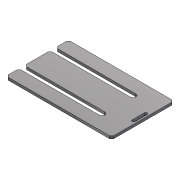
# Autodesk Inventor part: BC-10027
Saved by Autodesk Inventor 2016 (Build 200138000, 138)
## iProperties
Created: 2016-06-03
Part Number: BC-10027
Project: DIPOLO BC-3T- SIRIUS
Cost Center: 1504002005
Material: Aço Inox AISI 316
Document SubType Name: Modeling
Designer: reinaldo.basilio
Density: 7.85483 g/cm^3
Appearance: Semi-Polished
Description: Calço de ajuste da altura dos compensadores de gradiente.
Mass: 113.287 g
Surface Area: 128.736 cm^2
Volume: 14.4227 cm^3
RuleStatus: InUse
DocNumber: XXXXX-XXX-XXXX-00-001.ipt
Folder: .
Title: DIPOLO BC-3T- SIRIUS
Author: reinaldo.basilio
Autodesk Inventor part; units mm, degrees
ref_plane "YZ Plane" through (0, 0, 0) normal (1, 0, 0) x (0, 1, 0)
ref_plane "XZ Plane" through (0, 0, 0) normal (0, 1, 0) x (-1, 0, 0)
ref_plane "XY Plane" through (0, 0, 0) normal (0, 0, 1) x (1, 0, 0)
sketch "Sketch5" plane through (0, 0, 0) normal (0, 0, 1) x (1, 0, 0)
  line L0 (-31, 52.5) -> (31, 52.5)
  line L1 (31, 52.5) -> (31, -52.5)
  line L2 (-31, -52.5) -> (-31, 52.5)
  line L3 (-15.5, 27.5) -> (-15.5, -52.5) construction
  line L4 (-18.25, 27.5) -> (-18.25, -52.5)
  line L5 (-12.75, -52.5) -> (-12.75, 27.5)
  arc A0 (-12.75, 27.5) -> (-18.25, 27.5) centre (-15.5, 27.5) ccw
  arc A1 (-18.25, -52.5) -> (-12.75, -52.5) centre (-15.5, -52.5) ccw
  line L6 (0, 0) -> (0, 14.7878) construction
  line L7 (15.5, 27.5) -> (15.5, -52.5) construction
  line L8 (18.25, 27.5) -> (18.25, -52.5)
  line L9 (12.75, -52.5) -> (12.75, 27.5)
  arc A2 (18.25, 27.5) -> (12.75, 27.5) centre (15.5, 27.5) ccw
  arc A3 (12.75, -52.5) -> (18.25, -52.5) centre (15.5, -52.5) ccw
  line L10 (-18.25, -52.5) -> (-31, -52.5)
  line L11 (31, -52.5) -> (18.25, -52.5)
  line L12 (12.75, -52.5) -> (-12.75, -52.5)
  point P0 (0, 52.5)
  point P1 (-31, 0)
  point P2 (-15.5, -12.5)
  dimension "d8" = 62
  dimension "d9" = 105
  dimension "d10" = 15.5
  dimension "d11" = 5.5
  dimension "d12" = 80
  constraints: 30 end point, 8 point on circle, 6 symmetric about line, 5 parallel, 4 centre point, 4 perpendicular, 4 tangent, 3 midpoint, 1 horizontal, 1 horizontal alignment, 1 vertical, 1 vertical alignment, 2 other
  measures "d8" distance of L0.start L0.end
  measures "d9" distance of L2.start L0.start
  measures "d10" distance from line of L3 L6.start
  measures "d11" distance between parallel lines of L5 L4
  measures "d12" distance of L3.start L3.end
extrude "Extrusion5" add sketch "Sketch5" along normal blind 2.6 contours L0 L1 L11 L8 A2 L9 L12 L5 A0 L4 L10 L2
chamfer "Chamfer1" distance 2 angle 45 8 edges at (-18.25, -52.5, 1.3) (-12.75, -52.5, 1.3) (12.75, -52.5, 1.3) (18.25, -52.5, 1.3) (31, -52.5, 1.3) (-31, -52.5, 1.3) (31, 52.5, 1.3) (-31, 52.5, 1.3)
sketch "Sketch6" plane through (0, 0, 2.6) normal (0, 0, 1) x (1, 0, 0)
  line L0 (29, 52.5) -> (-29, 52.5) projected
  line L1 (6, 49.5) -> (-6, 49.5) construction
  line L2 (6, 51) -> (-6, 51)
  line L3 (-6, 48) -> (6, 48)
  arc A0 (6, 48) -> (6, 51) centre (6, 49.5) ccw
  arc A1 (-6, 51) -> (-6, 48) centre (-6, 49.5) ccw
  point P0 (0, 0)
  point P1 (0, 49.5)
  dimension "d18" = 12
  dimension "d19" = 3
  dimension "d20" = 1.5
  constraints: 8 end point, 4 point on circle, 4 tangent, 2 centre point, 1 horizontal, 1 midpoint, 1 parallel, 1 vertical alignment
  measures "d18" distance of L1.start L1.end
  measures "d19" distance between parallel lines of L0 L1
  measures "d20" radius of A0
extrude "Extrusion6" cut sketch "Sketch6" against normal through all
body "Solid5"
